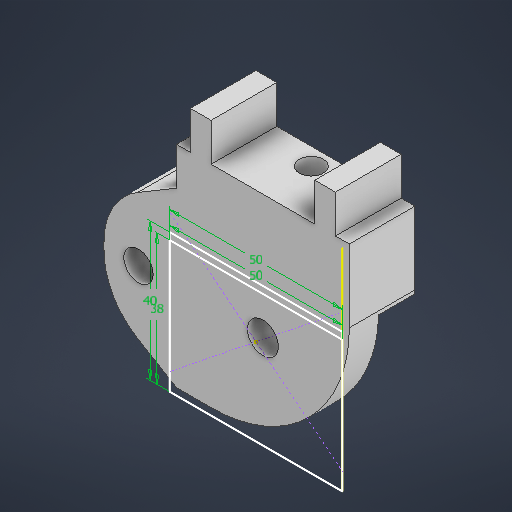
# Autodesk Inventor part: SuporteInferior
Saved by Autodesk Inventor 2026.1 (Build 301233000, 233)
## iProperties
Created: 2026-01-27
Part Number: SuporteInferior
Material: Generic
Document SubType Name: Modeling
Designer: fheli
Density: 1 g/cm^3
Appearance: Default
Author: fheli
Autodesk Inventor part; units mm, degrees
ref_plane "YZ Plane" through (0, 0, 0) normal (1, 0, 0) x (0, 1, 0)
ref_plane "XZ Plane" through (0, 0, 0) normal (0, 1, 0) x (-1, 0, 0)
ref_plane "XY Plane" through (0, 0, 0) normal (0, 0, 1) x (1, 0, 0)
sketch "Sketch1" plane through (0, 0, 0) normal (0, 0, 1) x (1, 0, 0)
  line L0 (-21, -21) -> (21, -21)
  line L1 (21, -21) -> (21, 21)
  line L2 (21, 21) -> (-21, 21)
  line L3 (-21, 21) -> (-21, -21)
  line L4 (-21, -21) -> (21, 21) construction
  line L5 (21, -21) -> (-21, 21) construction
  circle A0 centre (0, 0) radius 4.5
  circle A1 centre (-36, 0) radius 4.25
  line L6 (-46, 0) -> (-46, 12.5)
  line L7 (-46, 0) -> (-46, -12.5)
  line L8 (-25, -25) -> (25, -25)
  line L9 (25, -25) -> (25, 25)
  line L10 (-25, -25) -> (25, 25) construction
  line L11 (25, -25) -> (-25, 25) construction
  line L12 (-46, 12.5) -> (-25, 25)
  line L13 (-46, -12.5) -> (-25, -25)
  line L14 (0, 36) -> (15, 36)
  line L15 (15, 36) -> (15, 47)
  line L16 (15, 47) -> (21, 47)
  line L17 (21, 47) -> (21, 36)
  line L18 (21, 36) -> (25, 36)
  line L19 (25, 36) -> (25, 25)
  line L20 (0, 36) -> (-15, 36)
  line L21 (-15, 36) -> (-15, 47)
  line L22 (-15, 47) -> (-21, 47)
  line L23 (-21, 47) -> (-21, 36)
  line L24 (-21, 36) -> (-25, 36)
  line L25 (-25, 36) -> (-25, 25)
  line L26 (-25, 25) -> (25, 25)
  dimension "d0" = 42
  dimension "d1" = 42
  dimension "d2" = 9
  dimension "d5" = 8.5
  dimension "d6" = 46
  dimension "d10" = 50
  dimension "d12" = 15
  dimension "d14" = 6
  dimension "d15" = 11
  dimension "d21" = 11
  dimension "d22" = 50
  dimension "d23" = 25
  dimension "d24" = 4
  constraints: 54 end point, 5 perpendicular, 5 point on line, 4 horizontal, 4 midpoint, 3 vertical, 2 centre point, 2 parallel, 1 coincident
  measures "d0" distance of L2.end L1.end
  measures "d1" distance of L1.end L0.end
  measures "d2" diameter of A0
  measures "d5" diameter of A1
  measures "d6" distance of A0.centre L6.start
  measures "d10" distance of L9.end L8.end
  measures "d12" distance of L14.start L14.end
  measures "d14" distance of L15.end L16.end
  measures "d15" distance of L16.end L17.end
  measures "d21" distance of L11.end L24.end
  measures "d22" distance of L8.start L11.end
  measures "d23" distance of L7.end L6.end
  measures "d24" distance of L24.end L23.end
extrude "Extrusion1" add sketch "Sketch1" along normal blind 15 contours L3 L2 L1 L0 | L6 L12 L26 L9 L8 L13 L7 | L25 L24 L23 L22 L21 L20 L14 L15 L16 L17 L18 L19 L26
move faces "Move1" translate (0, 0, 10) faces at (0.1808, -18.1557, 15)
sketch "Sketch2" plane through (-25, -25, 25) normal (0, 0, 1) x (1, 0, 0)
  line L0 (0, 5) -> (50, 45) construction
  line L1 (50, 5) -> (0, 45) construction
  line L2 (50, 0) -> (50, 61) projected
  line L3 (50, 0) -> (0, 0)
  line L4 (0, 0) -> (0, 40)
  line L5 (0, 40) -> (50, 40)
  line L6 (50, 40) -> (50, 0)
  point P0 (25, 25)
  dimension "d32" = 50
  dimension "d33" = 40
  constraints: 12 end point, 2 midpoint, 2 parallel, 1 horizontal, 1 perpendicular
  measures "d32" distance of L4.end L5.end
  measures "d33" distance of L3.end L4.end
sketch "Sketch3" plane through (-25, -25, 25) normal (0, 0, 1) x (1, 0, 0)
  line L0 (50, 0) -> (50, 61) projected
  line L1 (50, 0) -> (0, 0)
  line L2 (0, 0) -> (0, 38)
  line L3 (0, 38) -> (50, 38)
  line L4 (50, 38) -> (50, 0)
  point P0 (25, 25)
  dimension "d34" = 50
  dimension "d35" = 38
  constraints: 8 end point, 2 parallel, 1 horizontal, 1 perpendicular
  measures "d34" distance of L2.end L3.end
  measures "d35" distance of L1.end L2.end
move faces "Move2" translate (0, 0, -2) faces at (18.1231, 4.0256, 25)
move faces "Move3" translate (0, 0, 4) faces at (18.1231, 4.0256, 0)
sketch "Sketch5" plane through (25, -25, 4) normal (0, 0, -1) x (-1, 0, 0)
  line L0 (0, 0) -> (0, 61) projected
  line L1 (0, 0) -> (50, 0)
  line L2 (50, 0) -> (50, 39)
  line L3 (50, 39) -> (0, 39)
  line L4 (0, 39) -> (0, 0)
  point P0 (25, 25)
  point P1 (0, 39)
  dimension "d48" = 50
  dimension "d49" = 39
  constraints: 8 end point, 2 parallel, 1 horizontal, 1 perpendicular
  measures "d48" distance of L3.end L2.end
  measures "d49" distance of L2.end L1.end
extrude "Extrusion4" cut sketch "Sketch5" against normal blind 10
sketch "Sketch6" plane through (-25, 14, 4) normal (0, -1, 0) x (1, 0, 0)
  circle A0 centre (25, 5) radius 3.5
  line L0 (50, 0) -> (0, 0) projected
  point P0 (25, -4)
  dimension "d52" = 7
  dimension "d53" = 5
  constraints: 1 centre point
  measures "d52" diameter of A0
  measures "d53" distance from line of L0 A0.centre
move faces "Move4" translate (0, 0, 0.5) faces at (0.1808, -18.1557, 14)
extrude "Extrusion5" cut sketch "Sketch6" against normal blind 30
fillet "Fillet1" radius 40 1 edges at (25, -25, 18.75)
fillet "Fillet2" radius 20 1 edges at (-46, -12.5, 13.5)
fillet "Fillet3" radius 20 1 edges at (-46, 12.5, 13.5)
body "Solid1"
